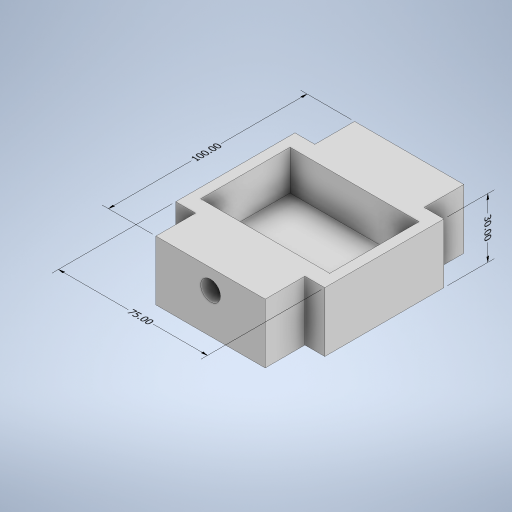
# Autodesk Inventor part: camera_support
Saved by Autodesk Inventor 2023 (Build 270158000, 158)
## iProperties
Created: 2022-07-04
Part Number: camera_support
Material: Genérico
Document SubType Name: Modeling
Designer: inigo
Density: 1 g/cm^3
Appearance: Valor por defecto
Author: inigo
Autodesk Inventor part; units mm, degrees
ref_plane "YZ Plane" through (0, 0, 0) normal (1, 0, 0) x (0, 1, 0)
ref_plane "XZ Plane" through (0, 0, 0) normal (0, 1, 0) x (-1, 0, 0)
ref_plane "XY Plane" through (0, 0, 0) normal (0, 0, 1) x (1, 0, 0)
sketch "Boceto1" plane through (0, 0, 0) normal (0, 1, 0) x (-1, 0, 0)
  line L0 (27.5, 50) -> (-27.5, 50)
  line L1 (-27.5, 50) -> (-27.5, -50)
  line L2 (-27.5, -50) -> (27.5, -50)
  line L3 (27.5, -50) -> (27.5, 50)
  line L4 (27.5, 50) -> (-27.5, -50) construction
  line L5 (-27.5, 50) -> (27.5, -50) construction
  point P0 (0, 0)
  dimension "d0" = 55
  dimension "d1" = 100
  constraints: 12 end point, 2 midpoint, 2 parallel, 1 horizontal, 1 perpendicular
  measures "d0" distance of L2.end L1.end
  measures "d1" distance of L1.end L0.end
extrude "Extrusión1" add sketch "Boceto1" along normal blind 30
sketch "Boceto3" plane through (-27.5, 0, 50) normal (0, 0, 1) x (1, 0, 0)
  circle A0 centre (27.5, 20) radius 5
  line L0 (0, 30) -> (55, 30) projected
  point P0 (27.5, 0)
  point P1 (27.5, 30)
  dimension "d10" = 10
  dimension "d11" = 10
  constraints: 1 centre point, 1 midpoint
  measures "d10" diameter of A0
  measures "d11" distance of point (27.5, 30) A0.centre
extrude "Extrusión3" cut sketch "Boceto3" against normal blind 15
sketch "Boceto9" plane through (0, 0, 0) normal (0, -1, 0) x (1, 0, 0)
  line L0 (-37.5, 30) -> (37.5, 30)
  line L1 (37.5, 30) -> (37.5, -30)
  line L2 (37.5, -30) -> (-37.5, -30)
  line L3 (-37.5, -30) -> (-37.5, 30)
  line L4 (-37.5, 30) -> (37.5, -30) construction
  line L5 (37.5, 30) -> (-37.5, -30) construction
  point P0 (0, 0)
  dimension "d52" = 75
  dimension "d53" = 60
  constraints: 12 end point, 2 midpoint, 2 parallel, 1 horizontal, 1 perpendicular
  measures "d52" distance of L1.end L2.end
  measures "d53" distance of L0.end L1.end
extrude "Extrusión7" add sketch "Boceto9" against normal blind 30
sketch "Boceto10" plane through (0, 30, 0) normal (0, 1, 0) x (1, 0, 0)
  line L0 (-32.5, 22.5) -> (32.5, 22.5)
  line L1 (32.5, 22.5) -> (32.5, -22.5)
  line L2 (32.5, -22.5) -> (-32.5, -22.5)
  line L3 (-32.5, -22.5) -> (-32.5, 22.5)
  line L4 (-32.5, 22.5) -> (32.5, -22.5) construction
  line L5 (32.5, 22.5) -> (-32.5, -22.5) construction
  point P0 (0, 0)
  dimension "d56" = 65
  dimension "d57" = 45
  constraints: 12 end point, 2 midpoint, 2 parallel, 1 horizontal, 1 perpendicular
  measures "d56" distance of L1.end L2.end
  measures "d57" distance of L0.end L1.end
extrude "Extrusión8" cut sketch "Boceto10" against normal blind 20
